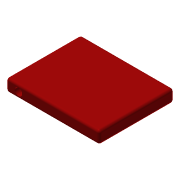
# Autodesk Inventor part: Tunel_Door
Saved by Autodesk Inventor 2016 (Build 200138000, 138)
## iProperties
Created: 2014-11-14
Part Number: Tunel_Door
Material: Polycarbonat, klar
Document SubType Name: Modeling
Designer: Gero Hofmann
Density: 1.2 g/cm^3
Appearance: Red
Author: Gero Hofmann
Autodesk Inventor part; units mm, degrees
ref_plane "YZ Plane" through (0, 0, 0) normal (1, 0, 0) x (0, 1, 0)
ref_plane "XZ Plane" through (0, 0, 0) normal (0, 1, 0) x (-1, 0, 0)
ref_plane "XY Plane" through (0, 0, 0) normal (0, 0, 1) x (1, 0, 0)
sketch "Skizze1" plane through (0, 0, 0) normal (0, 0, 1) x (1, 0, 0)
  line L0 (37.5, -30) -> (-37.5, -30)
  line L1 (-37.5, -30) -> (-37.5, 30)
  line L2 (-37.5, 30) -> (37.5, 30)
  line L3 (37.5, 30) -> (37.5, -30)
  line L4 (37.5, -30) -> (-37.5, 30) construction
  line L5 (-37.5, -30) -> (37.5, 30) construction
  point P0 (0, 0)
  dimension "d0" = 75
  dimension "d1" = 60
  constraints: 12 end point, 2 midpoint, 2 parallel, 1 horizontal, 1 perpendicular
  measures "d0" distance of L1.end L2.end
  measures "d1" distance of L0.end L1.end
extrude "Extrusion1" add sketch "Skizze1" along normal blind 10
hole "Bohrung1" at (-27.5, 30, 5) direction (0, -1, 0) diameter 6 depth 10 tip angle 118
mirror "Spiegeln1" about plane through (0, 0, 0) normal (0, 1, 0) of "Bohrung1"
hole "Bohrung2" at (-37.5, 27, 5) direction (1, 0, 0) diameter 2.459 end up to surface thread size "M3x0.5" class "6H" standard "ISO Metric profile"
fillet "Rundung2" radius 2 12 edges at (37.5, 0, 0) (37.5, 30, 5) (37.5, 0, 10) (37.5, -30, 5) (-37.5, 0, 0) (-37.5, -30, 5) (-37.5, 0, 10) (-37.5, 30, 5) (0, 30, 0) (0, 30, 10) (0, -30, 0) (0, -30, 10)
